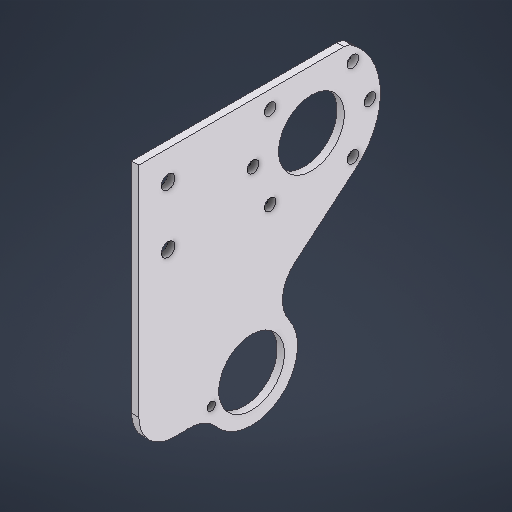
# Autodesk Inventor part: INSIDE_INTAKE_PLATE
Saved by Autodesk Inventor 2026.2 (Build 302298010, 298A)
## iProperties
Created: 2026-04-02
Part Number: INSIDE_INTAKE_PLATE
Material: Aluminum, 6061-T6
Document SubType Name: Sheet Metal
Designer: 4aida
Density: 2.71 g/cm^3
Sheet Metal Rule: Default_mm
Appearance: Metal-AL-6061 (Flat)
Mass: 78.9103 g
Surface Area: 208.249 cm^2
Volume: 29.1182 cm^3
Author: 4aida
Autodesk Inventor part; units mm, degrees
ref_plane "YZ Plane" through (0, 0, 0) normal (1, 0, 0) x (0, 1, 0)
ref_plane "XZ Plane" through (0, 0, 0) normal (0, 1, 0) x (-1, 0, 0)
ref_plane "XY Plane" through (0, 0, 0) normal (0, 0, 1) x (1, 0, 0)
sketch "Sketch1" plane through (0, 0, 0) normal (1, 0, 0) x (0, 1, 0)
  line L0 (-39.3892, -105) -> (-110, -20.8494)
  line L1 (-110, -20.8494) -> (-110, 0)
  line L2 (-110, 0) -> (0, 0)
  line L3 (0, 0) -> (0, -105)
  line L4 (0, -105) -> (-39.3892, -105)
  line L5 (-110, -20.8494) -> (-119.38, 0) construction
  line L6 (-119.38, 0) -> (-110, 0) construction
  line L7 (-50.8, -25.4) -> (0, -25.4) construction
  line L8 (0, -25.4) -> (0, 0) construction
  line L9 (0, 0) -> (-50.8, 0) construction
  line L10 (-50.8, 0) -> (-50.8, -25.4) construction
  line L11 (-50.8, -25.4) -> (0, 0) construction
  line L12 (0, -25.4) -> (-50.8, 0) construction
  circle A0 centre (-12.7, -12.7) radius 3
  circle A1 centre (-38.1, -12.7) radius 3
  circle A2 centre (-102.5, -49) radius 14.2875
  circle A3 centre (-25.4, -75) radius 14.2875
  circle A4 centre (-102.5, -49) radius 20
  circle A5 centre (-25.4, -75) radius 30
  line L13 (-50.8, -90.9637) -> (-50.8, -59.0363)
  line L14 (-102.5, -49) -> (-25.4, -75) construction
  point P0 (-25.4, -12.7)
  point P1 (-25.4, -25.4)
  point P2 (-103.1519, -29.0106)
  point P3 (-82.9275, -53.1131)
  point P4 (-50.8, -75)
  point P5 (-48.3813, -94.2836)
  point P6 (0, -90.9637)
  dimension "d0" = 50
  dimension "d1" = 119.38
  dimension "d2" = 50.8
  dimension "d3" = 25.4
  dimension "d4" = 25.4
  dimension "d5" = 12.7
  dimension "d6" = 6
  dimension "d7" = 6
  dimension "d8" = 28.575
  dimension "d9" = 102.5
  dimension "d10" = 49
  dimension "d13" = 110
  dimension "d16" = 60
  dimension "d17" = 25.4
  dimension "d18" = 25.4
  dimension "d20" = 40
  dimension "d44" = 81.3659
  measures "d0" angle of L0 L2
  measures "d1" distance from line of L3 L5.end
  measures "d2" distance of L7.start L7.end
  measures "d3" distance of L9.end L7.start
  measures "d4" distance of A1.centre A0.centre
  measures "d5" distance of point (-25.4, -12.7) A0.centre
  measures "d6" diameter of A0
  measures "d7" diameter of A1
  measures "d8" diameter of A2
  measures "d9" distance from line of A2.centre L3
  measures "d10" distance from line of L2 A2.centre
  measures "d13" distance between parallel lines of L3 L1
  measures "d16" diameter of A5
  measures "d17" distance from line of A3.centre L3
  measures "d18" distance of point (-50.8, -75) A3.centre
  measures "d20" diameter of A4
  measures "d44" distance of L14.start L14.end
extrude "Plate1" add sketch "Sketch1" along normal blind 3.175 contours L0 A4 L1 L2 L3 A5 | A5 L13 L3 | A4 L0 A2 | L0 A2 A4 | A5 L13
fillet "Corner Round1" radius 15 4 edges at (1.5875, -82.9275, -53.1131) (1.5875, -103.1519, -29.0106) (1.5875, -110, -20.8494) (1.5875, -110, 0)
fillet "Corner Round1" radius 6 1 edges at (1.5875, 0, -90.9637)
sketch "Sketch2" plane through (0, 0, 0) normal (-1, 0, 0) x (0, 0, 1)
  circle A0 centre (-31.4501, -106.5) radius 4.5847
  circle A1 centre (-49, -102.5) radius 14.2875 projected
  point P0 (0, 0)
  dimension "d21" = 9.1694
  dimension "d22" = 18
  dimension "d23" = 4
  constraints: 1 centre point
  measures "d21" diameter of A0
  measures "d22" distance of A1.centre A0.centre
  measures "d23" vertical distance of A0.centre A1.centre
hole "Hole1" at (0, -106.5, -31.4501) direction (1, 0, 0) diameter 3.683 end through all thread size "10-24 UNC" class "2B" standard "ANSI Unified Screw Threads"
sketch "Sketch3" plane through (3.175, 0, 0) normal (1, 0, 0) x (0, 0, -1)
  circle A0 centre (75, -25.4) radius 14.2875 projected
  circle A1 centre (75, -25.4) radius 25.4
  line L0 (49.6, -25.4) -> (100.4, -25.4)
  line L1 (92.9605, -7.4395) -> (57.0395, -7.4395)
  line L2 (75, -25.4) -> (57.0395, -7.4395)
  line L3 (92.9605, -43.3605) -> (57.0395, -43.3605)
  line L4 (75, -25.4) -> (92.9605, -43.3605)
  line L5 (25.4, -50.8) -> (0, -50.8)
  line L6 (0, -50.8) -> (0, 0)
  line L7 (0, 0) -> (25.4, 0)
  line L8 (25.4, 0) -> (25.4, -50.8)
  line L9 (25.4, -50.8) -> (0, 0) construction
  line L10 (0, -50.8) -> (25.4, 0) construction
  point P0 (12.7, -25.4)
  dimension "d31" = 50.8
  dimension "d32" = 45
  dimension "d40" = 25.4
  dimension "d41" = 50.8
  constraints: 22 end point, 6 coincident, 6 point on circle, 3 horizontal, 3 midpoint, 3 parallel, 1 centre point, 1 collinear, 1 horizontal alignment, 1 perpendicular, 1 point on line
  measures "d31" diameter of A1
  measures "d32" angle of L2 L0
  measures "d40" distance of L5.start L5.end
  measures "d41" distance of L7.end L5.start
hole "Hole2" at (3.175, -7.4395, -57.0395) at (3.175, -25.4, -49.6) at (3.175, -43.3605, -57.0395) at (3.175, -43.3605, -92.9605) at (3.175, -25.4, -100.4) at (3.175, -7.4395, -92.9605) direction (-1, 0, 0) diameter 5.105 end through all clearance for "Flat Head Machine Screw (82)" size "#10" standard "Ansi Unified Screw Threads"
equation "\"d5\" = 0.5 * d4"
equation "\"d7\" = d6"
equation "\"d29\" = Thickness"
equation "\"d14\" = Thickness"
equation "\"d18\" = d17"
equation "\"BendRadius\" = Thickness"
equation "\"BendReliefWidth\" = Thickness"
equation "\"BendReliefDepth\" = 0.5 * Thickness"
equation "\"CornerReliefSize\" = 4 * Thickness"
equation "\"MinimumRemnant\" = 2 * Thickness"
equation "\"TransitionRadius\" = BendRadius"
equation "\"JacobiRadiusSize\" = BendRadius"
equation "\"GapSize\" = Thickness"
equation "\"Thickness\" = 3.175"
body "Solid1"
